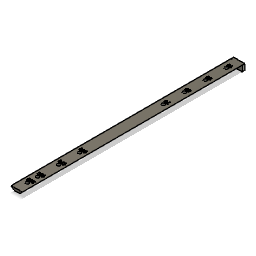
blind-joint-drill-guide-z-moddedZ-and-center v10 (Autodesk Fusion 360 design; units mm, degrees)
Autodesk Fusion 360 part; units mm, degrees
sketch "Sketch1" plane through (0, 0, 0) normal (0, 0, 1) x (1, 0, 0)
  line L0 (-2.875, 0) -> (2.875, 0)
  line L1 (-5.375, 2.5) -> (5.375, 2.5)
  line L2 (-5.375, 2.5) -> (-2.875, 0)
  line L3 (5.375, 2.5) -> (2.875, 0)
  line L4 (0, 7.9451) -> (0, -6.0549)
  dimension "d1" = 5.75
  dimension "d2" = 10.75
  dimension "d3" = 2.5
  constraint horizontal L0
  constraint horizontal L1
  constraint vertical L4
  constraint symmetric L1.start L1.end L4
  constraint symmetric L0.start L0.end L4
  constraint vertical origin L4.end
  constraint horizontal origin L0.start
  measures "d1" distance of L0.start L0.end
  measures "d2" distance of L1.start L1.end
  measures "d3" vertical distance of L0.start L1.start
extrude "Extrude1" add sketch "Sketch1" along normal blind 210
sketch "Sketch2" plane through (0, 0, 0) normal (0, 0, -1) x (-1, 0, 0)
  line L0 (2.875, 0) -> (5.375, 2.5)
  line L1 (5.375, 2.5) -> (-5.375, 2.5)
  line L2 (-5.375, 2.5) -> (-2.875, 0)
  line L3 (-2.875, 0) -> (2.875, 0)
  line L4 (-5.375, 2.5) -> (5.375, 2.5)
  line L5 (5.375, 2.5) -> (5.375, -3)
  line L6 (5.375, -3) -> (-5.375, -3)
  line L7 (-5.375, -3) -> (-5.375, 2.5)
  dimension "d6" = 10.75
  dimension "d7" = 5.5
  constraint horizontal L4
  constraint vertical L5
  constraint horizontal L6
  constraint vertical L7
  constraint coincident L1.end L2.start
  measures "d6" distance of L1.end L0.end
  measures "d7" distance of L1.end L6.end
extrude "Extrude2" add sketch "Sketch2" along normal blind 2.5
sketch "Sketch3" plane through (0, 0, 0) normal (0, -1, 0) x (1, 0, 0)
  line L0 (-2.875, 0) -> (2.875, 0)
  line L1 (2.875, 0) -> (2.875, 210)
  line L2 (2.875, 210) -> (-2.875, 210)
  line L3 (-2.875, 210) -> (-2.875, 0)
  circle A0 centre (0, 10) radius 1.5
  circle A1 centre (0, 170) radius 1.5
  circle A2 centre (0, 190) radius 1.5
  circle A3 centre (0, 200) radius 1.5
  circle A4 centre (0, 30) radius 1.5
  circle A5 centre (0, 50) radius 1.5
  circle A6 centre (0, 70) radius 1.5
  circle A7 centre (0, 150) radius 1.5
  dimension "d10" = 3
  dimension "d11" = 10
  dimension "d12" = 170
  dimension "d13" = 20
  dimension "d15" = 200
  dimension "d16" = 30
  dimension "d17" = 20
  dimension "d26" = 20
  dimension "d27" = 150
  constraint equal A1 A2
  constraint equal A0 A1
  constraint equal A1 A3
  constraint equal A4 A5
  constraint equal A0 A4
  constraint equal A5 A6
  constraint equal A6 A7
  measures "d10" diameter of A0
  measures "d11" distance of origin A0.centre
  measures "d12" distance of origin A1.centre
  measures "d13" distance of A1.centre A2.centre
  measures "d15" distance of origin A3.centre
  measures "d16" distance of origin A4.centre
  measures "d17" distance of A4.centre A5.centre
  measures "d26" distance of A5.centre A6.centre
  measures "d27" distance of origin A7.centre
extrude "Extrude3" cut sketch "Sketch3" against normal through all contours A0 | A1 | A2 | A3 | A4 | A5 | A6 | A7
sketch "Sketch5" plane through (0, 2.5, 0) normal (0, 1, 0) x (-1, 0, 0)
  circle A0 centre (0, 200) radius 1.5
  circle A1 centre (0, 10) radius 1.5
  circle A2 centre (0, 170) radius 1.5
  circle A3 centre (0, 70) radius 1.5
  circle A4 centre (0, 50) radius 1.5
  circle A5 centre (0, 190) radius 1.5
  circle A6 centre (0, 30) radius 1.5
  circle A7 centre (0, 150) radius 1.5
  line L0 (5.375, 0) -> (5.375, 210)
  line L1 (5.375, 210) -> (-5.375, 210)
  line L2 (-5.375, 210) -> (-5.375, 0)
  line L3 (-5.375, 0) -> (-5.375, -2.5)
  line L4 (-5.375, -2.5) -> (5.375, -2.5)
  line L5 (5.375, -2.5) -> (5.375, 0)
  line L6 (-3.1062, 5.2631) -> (3.1121, 5.2775) construction
  line L7 (3.1121, 5.2775) -> (3.1062, 7.8236) construction
  line L8 (3.1062, 7.8236) -> (-3.1121, 7.8091) construction
  line L9 (-3.1121, 7.8091) -> (-3.1062, 5.2631) construction
  line L10 (-3.1062, 25.2631) -> (3.1121, 25.2775) construction
  line L11 (3.1121, 25.2775) -> (3.1062, 27.8236) construction
  line L12 (3.1062, 27.8236) -> (-3.1121, 27.8091) construction
  line L13 (-3.1121, 27.8091) -> (-3.1062, 25.2631) construction
  line L14 (-3.1062, 45.2631) -> (3.1121, 45.2775) construction
  line L15 (3.1121, 45.2775) -> (3.1062, 47.8236) construction
  line L16 (3.1062, 47.8236) -> (-3.1121, 47.8091) construction
  line L17 (-3.1121, 47.8091) -> (-3.1062, 45.2631) construction
  line L18 (-3.1062, 65.2631) -> (3.1121, 65.2775) construction
  line L19 (3.1121, 65.2775) -> (3.1062, 67.8236) construction
  line L20 (3.1062, 67.8236) -> (-3.1121, 67.8091) construction
  line L21 (-3.1121, 67.8091) -> (-3.1062, 65.2631) construction
  line L22 (-3.1062, 145.2631) -> (3.1121, 145.2775) construction
  line L23 (3.1121, 145.2775) -> (3.1062, 147.8236) construction
  line L24 (3.1062, 147.8236) -> (-3.1121, 147.8091) construction
  line L25 (-3.1121, 147.8091) -> (-3.1062, 145.2631) construction
  line L26 (-3.1062, 165.2631) -> (3.1121, 165.2775) construction
  line L27 (3.1121, 165.2775) -> (3.1062, 167.8236) construction
  line L28 (3.1062, 167.8236) -> (-3.1121, 167.8091) construction
  line L29 (-3.1121, 167.8091) -> (-3.1062, 165.2631) construction
  line L30 (-3.1062, 185.2631) -> (3.1121, 185.2775) construction
  line L31 (3.1121, 185.2775) -> (3.1062, 187.8236) construction
  line L32 (3.1062, 187.8236) -> (-3.1121, 187.8091) construction
  line L33 (-3.1121, 187.8091) -> (-3.1062, 185.2631) construction
  line L34 (-3.1062, 195.2631) -> (3.1121, 195.2775) construction
  line L35 (3.1121, 195.2775) -> (3.1062, 197.8236) construction
  line L36 (3.1062, 197.8236) -> (-3.1121, 197.8091) construction
  line L37 (-3.1121, 197.8091) -> (-3.1062, 195.2631) construction
  dimension "d28" = 3
  dimension "d29" = 3
  dimension "d30" = 3
  dimension "d31" = 3
  dimension "d32" = 3
  dimension "d33" = 3
  dimension "d34" = 3
  dimension "d35" = 3
  text T0 "10" font "Arial" height 3 bold align centre middle in box 6.2183 x 2.5461 at (-3.1062, 5.2631) x (0.999997, 0.002326) y (-0.002326, 0.999997) spacing 1
  text T1 "30" font "Arial" height 3 bold align centre middle in box 6.2183 x 2.5461 at (-3.1062, 25.2631) x (0.999997, 0.002326) y (-0.002326, 0.999997) spacing 1
  text T2 "50" font "Arial" height 3 bold align centre middle in box 6.2183 x 2.5461 at (-3.1062, 45.2631) x (0.999997, 0.002326) y (-0.002326, 0.999997) spacing 1
  text T3 "70" font "Arial" height 3 bold align centre middle in box 6.2183 x 2.5461 at (-3.1062, 65.2631) x (0.999997, 0.002326) y (-0.002326, 0.999997) spacing 1
  text T4 "150" font "Arial" height 3 bold align centre middle in box 6.2183 x 2.5461 at (-3.1062, 145.2631) x (0.999997, 0.002326) y (-0.002326, 0.999997) spacing 1
  text T5 "170" font "Arial" height 3 bold align centre middle in box 6.2183 x 2.5461 at (-3.1062, 165.2631) x (0.999997, 0.002326) y (-0.002326, 0.999997) spacing 1
  text T6 "190" font "Arial" height 3 bold align centre middle in box 6.2183 x 2.5461 at (-3.1062, 185.2631) x (0.999997, 0.002326) y (-0.002326, 0.999997) spacing 1
  text T7 "200" font "Arial" height 3 bold align centre middle in box 6.2183 x 2.5461 at (-3.1062, 195.2631) x (0.999997, 0.002326) y (-0.002326, 0.999997) spacing 1
extrude "Extrude6" cut sketch "Sketch5" against normal blind 0.6 text T5 T6 T7 T4 T3 T2 T1 T0
